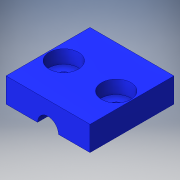
# Autodesk Inventor part: TopOfSquareSupport
Saved by Autodesk Inventor 2016 SP1 (Build 200210100, 210)
## iProperties
Created: 2015-12-11
Part Number: TopOfSquareSupport
Material: PC/ABS Plastic
Document SubType Name: Modeling
Designer: steele
Density: 0.357273 g/cm^3
Appearance: Blue - Wall Paint - Glossy
Author: steele
Autodesk Inventor part; units mm, degrees
ref_plane "YZ Plane" through (0, 0, 0) normal (1, 0, 0) x (0, 1, 0)
ref_plane "XZ Plane" through (0, 0, 0) normal (0, 1, 0) x (-1, 0, 0)
ref_plane "XY Plane" through (0, 0, 0) normal (0, 0, 1) x (1, 0, 0)
sketch "Sketch5" plane through (0, 0, 0) normal (0, 1, 0) x (-1, 0, 0)
  line L0 (-19.05, 19.05) -> (-19.05, -19.05)
  line L1 (-19.05, -19.05) -> (19.05, -19.05)
  line L2 (19.05, -19.05) -> (19.05, 19.05)
  line L3 (19.05, 19.05) -> (-19.05, 19.05)
  line L4 (-19.05, 19.05) -> (19.05, -19.05) construction
  line L5 (-19.05, -19.05) -> (19.05, 19.05) construction
  point P0 (0, 0)
  dimension "d23" = 38.1
  constraints: 12 end point, 2 midpoint, 2 parallel, 2 perpendicular, 1 vertical
  measures "d23" distance of L0.start L0.end
extrude "Extrusion3" add sketch "Sketch5" along normal blind 11.1125
sketch "Sketch6" plane through (-19.05, 0, 19.05) normal (0, 0, 1) x (1, 0, 0)
  point P0 (19.05, 0)
  point P1 (19.05, 0)
  constraints: 1 coincident
hole "Hole2" at (0, 0, 19.05) direction (0, 0, -1) diameter 9.525 end through all
sketch "Sketch7" plane through (0, 11.1125, 0) normal (0, 1, 0) x (1, 0, 0)
  line L0 (-19.05, 19.05) -> (-19.05, -19.05) projected
  line L1 (19.05, -19.05) -> (19.05, 19.05) projected
  point P0 (0, 0)
  point P1 (-11.9062, 0)
  point P2 (11.9062, 0)
  dimension "d33" = 7.1437
  dimension "d34" = 7.1437
  measures "d33" distance from line of point (-11.906, 0) L0
  measures "d34" distance from line of point (11.906, 0) L1
hole "Hole3" at (-11.9062, 11.1125, 0) at (11.9062, 11.1125, 0) direction (0, -1, 0) diameter 13.335 depth 6.096
sketch "Sketch8" plane through (0, 11.1125, 0) normal (0, 1, 0) x (1, 0, 0)
  line L0 (-19.05, 19.05) -> (-19.05, -19.05) projected
  line L1 (19.05, -19.05) -> (19.05, 19.05) projected
  point P0 (0, 0)
  point P1 (-11.9062, 0)
  point P2 (11.9062, 0)
  dimension "d42" = 7.1437
  dimension "d43" = 7.1437
  measures "d42" distance from line of point (-11.906, 0) L0
  measures "d43" distance from line of L1 point (11.906, 0)
hole "Hole4" at (-11.9062, 11.1125, 0) at (11.9062, 11.1125, 0) direction (0, -1, 0) diameter 5.1054 end through all clearance for "Flat Head Machine Screw (82)" size "#10" standard "Ansi Unified Screw Threads"
equation "\"d23\" = width"
equation "\"d24\" = heightOfTopSection"
equation "\"d26\" = topHoleDiam"
equation "\"d33\" = edgeToBoltHole"
equation "\"d34\" = edgeToBoltHole"
equation "\"d35\" = washerDiam"
equation "\"d40\" = depthForSocketHead"
equation "\"d42\" = edgeToBoltHole"
equation "\"d43\" = edgeToBoltHole"
equation "\"bottomHoleDiam\" = 9.525"
equation "\"width\" = 38.1"
equation "\"deltaBottomToTop\" = 25.4"
equation "\"d0\" = width"
equation "\"d1\" = heightOfBottomHole"
equation "\"d2\" = 0"
equation "\"d3\" = bottomHoleDiam"
equation "\"d5\" = 0"
equation "\"topHoleDiam\" = 9.525"
equation "\"height\" = deltaBottomToTop + heightOfBottomHole + heightOfTopHole"
equation "\"heightOfTopSection\" = heightOfBottomHole"
equation "\"edgeToBoltHole\" = -0.25 * bottomHoleDiam + 0.25 * width"
equation "\"washerDiam\" = 13.335"
equation "\"depthForSocketHead\" = 6.096"
equation "\"heightOfTopSupport\" = 12.7"
equation "\"heightOfBottomHole\" = 11.1125"
equation "\"heightOfTopHole\" = 11.1125"
body "Solid2"
